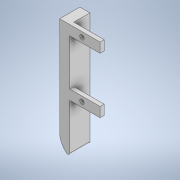
# Autodesk Inventor part: first joint
Saved by Autodesk Inventor 2022 (Build 260153000, 153)
## iProperties
Created: 2023-07-22
Part Number: first joint
Material: Generic
Document SubType Name: Modeling
Designer: Eric Cao
Density: 1 g/cm^3
Appearance: Default
Author: Eric Cao
Autodesk Inventor part; units mm, degrees
ref_plane "YZ Plane" through (0, 0, 0) normal (1, 0, 0) x (0, 1, 0)
ref_plane "XZ Plane" through (0, 0, 0) normal (0, 1, 0) x (-1, 0, 0)
ref_plane "XY Plane" through (0, 0, 0) normal (0, 0, 1) x (1, 0, 0)
sketch "Sketch1" plane through (0, 0, 0) normal (0, 0, 1) x (1, 0, 0)
  line L0 (0, 34.8483) -> (20, 34.8483)
  line L1 (20, 34.8483) -> (20, 29.9983)
  line L2 (0, 34.8483) -> (0, 0)
  line L3 (20, 29.9983) -> (5, 29.9983)
  line L4 (5, 29.9983) -> (5, 7.1983)
  line L5 (5, 7.1983) -> (20, 7.1983)
  line L6 (20, 7.1983) -> (20, 2.3483)
  line L7 (20, 2.3483) -> (5, 2.3483)
  line L8 (0, 0) -> (0, -15.1517)
  line L9 (5, -15.1517) -> (5, 2.3483)
  line L10 (5, -15.1517) -> (5, -22.2152)
  arc A0 (0, -15.1517) -> (5, -22.2152) centre (9.8436, -13.4852) ccw
  dimension "d14" = 20
  dimension "d15" = 4.85
  dimension "d17" = 4.85
  dimension "d18" = 22.8
  dimension "d19" = 20
  dimension "d20" = 5
  dimension "d22" = 9.9837
  dimension "d23" = 90
  dimension "d24" = 29.9983
  dimension "d25" = 10.1564
  dimension "d26" = 43.4835
  dimension "d27" = 45.15
  constraints: 22 end point, 5 perpendicular, 3 vertical, 2 horizontal, 2 point on circle, 1 centre point, 1 point on line
  measures "d14" distance of L0.start L0.end
  measures "d15" distance of L0.end L1.end
  measures "d17" distance of L5.end L6.end
  measures "d18" distance of L3.end L4.end
  measures "d19" distance between parallel lines of L6 L8
  measures "d20" distance between parallel lines of L2 L4
  measures "d22" radius of A0
  measures "d23" angle of L9 L3
  measures "d24" distance from line of L2.end L3
  measures "d25" distance from line of A0.centre L1
  measures "d26" distance from line of A0.centre L3
  measures "d27" distance from line of L9.start L3
extrude "Extrusion1" add sketch "Sketch1" against normal blind 10
sketch "Sketch2" plane through (20, 29.9983, 0) normal (1, 0, 0) x (0, 0, -1)
  line L0 (0, 0) -> (10, 0) projected
  line L1 (2, 0) -> (2, 4.85)
  line L2 (0, 4.85) -> (10, 4.85) projected
  line L3 (2, 4.85) -> (10, 4.85)
  line L4 (10, 4.85) -> (10, 0)
  line L5 (10, -45.15) -> (10, 4.85) projected
  line L6 (0, 0) -> (0, 4.85) projected
  line L7 (0, 0) -> (10, 0) projected
  line L8 (2, 0) -> (10, 0)
  line L9 (10, -22.8) -> (10, -27.65) projected
  line L10 (2, -27.65) -> (2, -22.8)
  line L11 (2, -22.8) -> (10, -22.8)
  line L12 (10, -22.8) -> (10, -27.65)
  line L13 (2, -27.65) -> (10, -27.65)
  point P0 (0, -29.9983)
  point P1 (10, -11.4)
  dimension "d30" = 2
  dimension "d33" = 11.4
  dimension "d36" = 27.65
  constraints: 16 end point, 3 point on line, 2 vertical, 1 collinear, 1 perpendicular, 9 other
  measures "d30" distance between parallel lines of L6 L1
  measures "d33" distance of L0.end point (10, -11.4)
  measures "d36" distance of L1.start L10.start
extrude "Extrusion2" cut sketch "Sketch2" against normal blind 15 contours L5 L13 L10 L11 | L1 L2 L4 L0
fillet "Fillet1" radius 1 1 edges at (5, -22.2152, -5)
sketch "Sketch3" plane through (0, 0, 0) normal (0, 0, 1) x (1, 0, 0)
  line L0 (20, 34.8483) -> (0, 34.8483) projected
  line L1 (5, 7.1983) -> (5, 29.9983) projected
  circle A0 centre (11.05, 32.4233) radius 1.1
  circle A1 centre (11.05, 4.7733) radius 1.1
  point P0 (0, 0)
  dimension "d42" = 2.425
  dimension "d43" = 6.05
  dimension "d44" = 1.1
  dimension "d47" = 27.65
  constraints: 2 centre point, 1 coincident, 1 vertical, 2 other
  measures "d42" distance from line of L0 point (11.05, 32.423)
  measures "d43" distance from line of L1 point (11.05, 32.423)
  measures "d44" radius of A0
  measures "d47" distance of A0.centre A1.centre
extrude "Extrusion3" cut sketch "Sketch3" against normal blind 15
body "Solid1"
